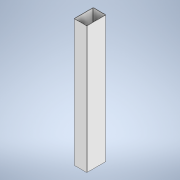
# Autodesk Inventor part: tubo3-40x80x800
Saved by Autodesk Inventor 2021 (Build 250183000, 183)
## iProperties
Created: 2026-05-19
Part Number: tubo3-40x80x800
Material: Acero, carbono
Document SubType Name: Modeling
Designer: nelso
Density: 7.85 g/cm^3
Appearance: Blanco
Author: nelso
Autodesk Inventor part; units mm, degrees
ref_plane "YZ Plane" through (0, 0, 0) normal (1, 0, 0) x (0, 1, 0)
ref_plane "XZ Plane" through (0, 0, 0) normal (0, 1, 0) x (-1, 0, 0)
ref_plane "XY Plane" through (0, 0, 0) normal (0, 0, 1) x (1, 0, 0)
sketch "Sketch2" plane through (0, 0, 0) normal (0, 1, 0) x (-1, 0, 0)
  line L0 (-40, 60) -> (40, 60)
  line L1 (40, 60) -> (40, -60)
  line L2 (40, -60) -> (-40, -60)
  line L3 (-40, -60) -> (-40, 60)
  line L4 (-40, 60) -> (40, -60) construction
  line L5 (40, 60) -> (-40, -60) construction
  line L6 (-37.76, 57.76) -> (37.76, 57.76)
  line L7 (37.76, 57.76) -> (37.76, -57.76)
  line L8 (37.76, -57.76) -> (-37.76, -57.76)
  line L9 (-37.76, -57.76) -> (-37.76, 57.76)
  line L10 (-37.76, 57.76) -> (37.76, -57.76) construction
  line L11 (37.76, 57.76) -> (-37.76, -57.76) construction
  point P0 (0, 0)
  dimension "d8" = 80
  dimension "d9" = 120
  dimension "d10" = 75.52
  dimension "d61" = 115.52
  constraints: 24 end point, 4 midpoint, 4 parallel, 2 horizontal, 2 perpendicular
  measures "d8" distance of L1.end L2.end
  measures "d9" distance of L0.end L1.end
  measures "d10" distance of L7.end L8.end
  measures "d61" distance of L6.end L7.end
extrude "Extrusion2" add sketch "Sketch2" along normal mid plane 790
fillet "Fillet2" radius 4 4 edges at (-40, 0, 60) (40, 0, 60) (40, 0, -60) (-40, 0, -60)
fillet "Fillet2" radius 2 4 edges at (37.76, 0, 57.76) (-37.76, 0, -57.76) (37.76, 0, -57.76) (-37.76, 0, 57.76)
body "Solid2"
